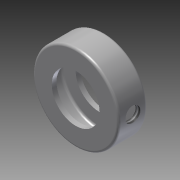
# Autodesk Inventor part: Misc_ShaftCollar_Triangle_SC10
Saved by Autodesk Inventor 2013 (Build 170138000, 138)
## iProperties
Category: Miscellaneous
Company: Autodesk Inc.
Created: 2012-12-03
Part Number: Misc_ShaftCollar_Triangle_SC10
Document SubType Name: Modeling
Designer: Autodesk Inc.
Density: 1 g/cm^3
Material: Generic
Author: Autodesk Inc.
Autodesk Inventor part; units mm, degrees
ref_plane "XZ Plane" through (0, 0, 0) normal (0, 1, 0) x (-1, 0, 0)
ref_plane "XY Plane" through (0, 0, 0) normal (0, 0, 1) x (1, 0, 0)
sketch "Sketch1" plane through (0, 0, 0) normal (0, 0, 1) x (1, 0, 0)
  circle A0 centre (0, 0) radius 14.2875
  dimension "d0" = 28.575
  constraints: 1 centre point, 1 coincident
  measures "d0" diameter of A0
extrude "Extrusion1" add sketch "Sketch1" along normal mid plane 9.525
fillet "Fillet1" radius 0.7937 2 edges at (-14.2875, 0, 4.7625) (-14.2875, 0, -4.7625)
sketch "Sketch2" plane through (0, 0, 4.7625) normal (0, 0, 1) x (1, 0, 0)
  circle A0 centre (0, 0) radius 13.4938 projected
  circle A1 centre (0, 0) radius 7.9375
  dimension "d4" = 15.875
  constraints: 1 centre point, 1 coincident
  measures "d4" diameter of A1
extrude "Extrusion2" cut sketch "Sketch2" against normal up to next contours A1
sketch "Sketch3" plane through (0, 0, 0) normal (1, 0, 0) x (0, 1, 0)
  line L0 (7.9375, 3.175) -> (11.9062, 3.175)
  line L1 (12.7, 2.3813) -> (12.7, -2.3813)
  line L2 (11.9062, -3.175) -> (7.9375, -3.175)
  line L3 (7.9375, -3.175) -> (7.9375, 3.175)
  line L4 (-13.4938, 4.7625) -> (13.4938, 4.7625) projected
  line L5 (13.4938, -4.7625) -> (-13.4938, -4.7625) projected
  line L6 (14.2875, -3.9688) -> (14.2875, 3.9688) projected
  line L7 (7.9375, 4.7625) -> (7.9375, -4.7625) projected
  arc A0 (12.7, 2.3813) -> (11.9062, 3.175) centre (11.9062, 2.3813) ccw
  arc A1 (11.9062, -3.175) -> (12.7, -2.3813) centre (11.9062, -2.3813) ccw
  line L8 (0, 4.7625) -> (0, -4.7625)
  point P0 (0, 0)
  dimension "d7" = 1.5875
  dimension "d8" = 1.5875
  dimension "d9" = 1.5875
  dimension "d10" = 0.7937
  constraints: 10 end point, 4 point on circle, 4 tangent, 2 centre point, 2 midpoint, 2 parallel, 1 collinear, 1 equal radius, 1 horizontal, 1 perpendicular
  measures "d7" distance between parallel lines of L4 L0
  measures "d8" distance between parallel lines of L5 L2
  measures "d9" distance between parallel lines of L6 L1
  measures "d10" radius of A0
revolve "Revolution1" cut sketch "Sketch3" angle 360 about axis through (0, 0, 4.7625) along (0, 0, -1) contours L0 A0 L1 A1 L2 L3
ref_plane "Work Plane1" through (14.2875, 0, 0) normal (1, 0, 0) x (0, 1, 0)
sketch "Sketch4" plane through (14.2875, 0, 0) normal (1, 0, 0) x (0, 1, 0)
  line L0 (13.4938, -4.7625) -> (-13.4937, -4.7625) projected
  line L1 (14.2875, -3.9688) -> (14.2875, 3.9688) projected
  point P0 (0, 0)
  point P1 (0, 0)
  constraints: 1 coincident
hole "Hole1" at (14.2875, 0, 0) direction (-1, 0, 0) diameter 4.9784 depth 25.4 tip angle 118 thread size "1/4-20 UNC" class "2B" standard "ANSI Unified Screw Threads"
equation "\"d8\" = d7"
equation "\"d9\" = d7"
body "Solid1"
